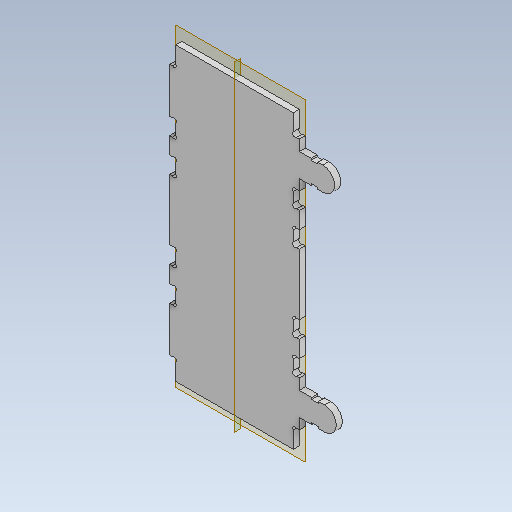
# Autodesk Inventor part: cover
Saved by Autodesk Inventor 2020 (Build 240168000, 168)
## iProperties
Created: 2019-12-17
Part Number: cover
Material: Generic
Document SubType Name: Modeling
Designer: erwin
Density: 1 g/cm^3
Appearance: Default
Author: erwin
Autodesk Inventor part; units mm, degrees
ref_plane "YZ Plane" through (0, 0, 0) normal (1, 0, 0) x (0, 1, 0)
ref_plane "XZ Plane" through (0, 0, 0) normal (0, 1, 0) x (-1, 0, 0)
ref_plane "XY Plane" through (0, 0, 0) normal (0, 0, 1) x (1, 0, 0)
ref_plane "Work Plane1" through (0, 0, 0) normal (0, 0, 1) x (1, 0, 0)
sketch "Sketch1" plane through (0, 0, 0) normal (0, 0, 1) x (1, 0, 0)
  line L0 (-35, -85) -> (-35, 85) projected
  line L1 (35, -85) -> (-35, -85) projected
  line L2 (35, 85) -> (35, -85) projected
  line L3 (-35, 85) -> (35, 85) projected
  line L4 (38.6, -88.6) -> (-38.6, -88.6)
  line L5 (-38.6, -88.6) -> (-38.6, 88.6)
  line L6 (-38.6, 88.6) -> (38.6, 88.6)
  line L7 (52.6163, 61.6) -> (37.6163, 61.6) construction
  arc A0 (52.6163, 54.6) -> (52.6163, 68.6) centre (52.6163, 61.6) ccw
  line L8 (38.6, -61.6) -> (53.6, -61.6) construction
  arc A1 (53.6, -68.6) -> (53.6, -54.6) centre (53.6, -61.6) ccw
  line L9 (38.6, 88.6) -> (38.6, 68.6)
  line L10 (38.6, 54.6) -> (38.6, -54.6)
  line L11 (38.6, -68.6) -> (38.6, -88.6)
  line L12 (45.6, 68.6) -> (45.6, 67.6)
  line L13 (45.6, 67.6) -> (49.6, 67.6)
  line L14 (49.6, 67.6) -> (49.6, 68.6)
  line L15 (49.6, 54.6) -> (49.6, 55.6)
  line L16 (49.6, 55.6) -> (45.6, 55.6)
  line L17 (45.6, 55.6) -> (45.6, 54.6)
  line L18 (38.6, 54.6) -> (45.6, 54.6)
  line L19 (49.6, 54.6) -> (52.6163, 54.6)
  line L20 (52.6163, 68.6) -> (49.6, 68.6)
  line L21 (45.6, 68.6) -> (38.6, 68.6)
  line L22 (49.9959, -54.6) -> (49.9945, -55.6)
  line L23 (49.9945, -55.6) -> (45.9945, -55.6)
  line L24 (45.9945, -55.6) -> (45.9959, -54.6)
  line L25 (49.9761, -68.6) -> (49.9736, -67.6)
  line L26 (49.9736, -67.6) -> (45.9736, -67.6)
  line L27 (45.9736, -67.6) -> (45.9761, -68.6)
  line L28 (53.6, -54.6) -> (49.9959, -54.6)
  line L29 (45.9959, -54.6) -> (38.6, -54.6)
  line L30 (38.6, -68.6) -> (45.9761, -68.6)
  line L31 (49.9761, -68.6) -> (53.6, -68.6)
  point P0 (0, 0)
  dimension "d1" = 7
  dimension "d2" = 7
  dimension "d7" = 4
  dimension "d8" = 1
  dimension "d9" = 7
  dimension "d10" = 15
  dimension "d11" = 15
  dimension "d12" = 3.6
  dimension "d13" = 3.6
  dimension "d14" = 1
  dimension "d15" = 1
  dimension "d16" = 20
  dimension "d17" = 20
  constraints: 60 end point, 14 parallel, 9 perpendicular, 8 tangent, 6 equal length, 5 point on circle, 3 collinear, 2 centre point, 2 point on line, 2 other
  measures "d1" radius of A0
  measures "d2" radius of A1
  measures "d7" distance of L12.end L13.end
  measures "d8" distance of L13.end L14.end
  measures "d9" distance between parallel lines of L9 L12
  measures "d10" distance of L7.start L7.end
  measures "d11" distance of L8.start L8.end
  measures "d12" distance between parallel lines of L2 L10
  measures "d13" distance between parallel lines of L6 L3
  measures "d14" distance of L22.start L22.end
  measures "d15" distance of L25.end L25.start
  measures "d16" distance between parallel lines of L4 L30
  measures "d17" distance between parallel lines of L6 L21
extrude "Extrusion1" add sketch "Sketch1" along normal blind 3.6 contours L0 L3 L2 L1 | L4 L5 L6 L9 L21 L12 L13 L14 L20 A0 L19 L15 L16 L17 L18 L10 L29 L24 L23 L22 L28 A1 L31 L25 L26 L27 L30 L11
sketch "Sketch2" plane through (0, 0, 0) normal (0, 0, -1) x (-1, 0, 0)
  line L0 (-49.6, 67.6) -> (-45.6, 67.6) projected
  line L1 (-49.6, 68.6) -> (-49.6, 67.6) projected
  line L2 (-52.6163, 68.6) -> (-49.6, 68.6) projected
  arc A0 (-52.6163, 68.6) -> (-52.6163, 54.6) centre (-52.6163, 61.6) ccw projected
  line L3 (-49.6, 54.6) -> (-52.6163, 54.6) projected
  line L4 (-49.6, 55.6) -> (-49.6, 54.6) projected
  line L5 (-45.6, 55.6) -> (-49.6, 55.6) projected
  line L6 (-45.6, 54.6) -> (-45.6, 55.6) projected
  line L7 (-38.6, 54.6) -> (-45.6, 54.6) projected
  line L8 (-38.6, -54.6) -> (-38.6, 54.6) projected
  line L9 (-45.9959, -54.6) -> (-38.6, -54.6) projected
  line L10 (-45.9945, -55.6) -> (-45.9959, -54.6) projected
  line L11 (-49.9945, -55.6) -> (-45.9945, -55.6) projected
  line L12 (-49.9959, -54.6) -> (-49.9945, -55.6) projected
  line L13 (-53.6, -54.6) -> (-49.9959, -54.6) projected
  arc A1 (-53.6, -54.6) -> (-53.6, -68.6) centre (-53.6, -61.6) ccw projected
  line L14 (-49.9761, -68.6) -> (-53.6, -68.6) projected
  line L15 (-49.9736, -67.6) -> (-49.9761, -68.6) projected
  line L16 (-45.9736, -67.6) -> (-49.9736, -67.6) projected
  line L17 (-45.9761, -68.6) -> (-45.9736, -67.6) projected
  line L18 (-38.6, -68.6) -> (-45.9761, -68.6) projected
  line L19 (-38.6, -88.6) -> (-38.6, -68.6) projected
  line L20 (38.6, -88.6) -> (-38.6, -88.6) projected
  line L21 (38.6, 88.6) -> (38.6, -88.6) projected
  line L22 (-38.6, 88.6) -> (38.6, 88.6) projected
  line L23 (-38.6, 68.6) -> (-38.6, 88.6) projected
  line L24 (-45.6, 68.6) -> (-38.6, 68.6) projected
  line L25 (-45.6, 67.6) -> (-45.6, 68.6) projected
  line L26 (35, -85) -> (35, 85) projected
  line L27 (35, 85) -> (-35, 85) projected
  line L28 (-35, 85) -> (-35, -85) projected
  line L29 (-35, -85) -> (35, -85) projected
  line L30 (38.6, 88.6) -> (38.6, -88.6) projected
  line L31 (-38.6, -88.6) -> (38.6, -88.6)
  line L32 (38.6, -88.6) -> (38.6, -85)
  line L33 (38.6, -85) -> (-38.6, -85)
  line L34 (-38.6, -85) -> (-38.6, -88.6)
  line L35 (-38.6, -85) -> (-35, -85)
  line L36 (-35, -85) -> (-35, -75)
  line L37 (-35, -75) -> (-38.6, -75)
  line L38 (-38.6, -75) -> (-38.6, -85)
  line L39 (-38.6, -54.6) -> (-38.6, 54.6) projected
  line L40 (-38.6, -48.2) -> (-35, -48.2)
  line L41 (-35, -48.2) -> (-35, -38.2)
  line L42 (-35, -38.2) -> (-38.6, -38.2)
  line L43 (-38.6, -38.2) -> (-38.6, -48.2)
  line L44 (-35, -28.2) -> (-38.6, -28.2)
  line L45 (-38.6, -28.2) -> (-38.6, -38.2)
  line L46 (-38.6, -38.2) -> (-35, -38.2)
  line L47 (-35, -38.2) -> (-35, -28.2)
  line L48 (-35, -18.2) -> (-38.6, -18.2)
  line L49 (-38.6, -18.2) -> (-38.6, -28.2)
  line L50 (-38.6, -28.2) -> (-35, -28.2)
  line L51 (-35, -28.2) -> (-35, -18.2)
  line L52 (-38.6, 0) -> (49.1643, 0) construction
  line L53 (-38.6, 88.6) -> (-38.6, 68.6)
  line L54 (38.6, 88.6) -> (-38.6, 88.6)
  line L55 (-35, 85) -> (35, 85)
  line L56 (-38.6, 88.6) -> (38.6, 88.6)
  line L57 (38.6, 88.6) -> (38.6, 85)
  line L58 (38.6, 85) -> (-38.6, 85)
  line L59 (-38.6, 85) -> (-38.6, 88.6)
  line L60 (-38.6, 85) -> (-35, 85)
  line L61 (-35, 85) -> (-35, 75)
  line L62 (-35, 75) -> (-38.6, 75)
  line L63 (-38.6, 75) -> (-38.6, 85)
  line L64 (-38.6, 48.2) -> (-35, 48.2)
  line L65 (-35, 48.2) -> (-35, 38.2)
  line L66 (-35, 38.2) -> (-38.6, 38.2)
  line L67 (-38.6, 38.2) -> (-38.6, 48.2)
  line L68 (-35, 28.2) -> (-38.6, 28.2)
  line L69 (-38.6, 28.2) -> (-38.6, 38.2)
  line L70 (-38.6, 38.2) -> (-35, 38.2)
  line L71 (-35, 38.2) -> (-35, 28.2)
  line L72 (-35, 18.2) -> (-38.6, 18.2)
  line L73 (-38.6, 18.2) -> (-38.6, 28.2)
  line L74 (-38.6, 28.2) -> (-35, 28.2)
  line L75 (-35, 28.2) -> (-35, 18.2)
  line L76 (38.6, -88.6) -> (-38.6, -88.6) construction
  line L77 (0, -88.6) -> (0, 88.6) construction
  line L78 (38.6, -54.6) -> (38.6, 54.6)
  line L79 (35, 85) -> (35, -85)
  line L80 (38.6, -85) -> (35, -85)
  line L81 (35, -85) -> (35, -75)
  line L82 (35, -75) -> (38.6, -75)
  line L83 (38.6, -75) -> (38.6, -85)
  line L84 (38.6, -54.6) -> (38.6, 54.6)
  line L85 (38.6, -48.2) -> (35, -48.2)
  line L86 (35, -48.2) -> (35, -38.2)
  line L87 (35, -38.2) -> (38.6, -38.2)
  line L88 (38.6, -38.2) -> (38.6, -48.2)
  line L89 (35, -28.2) -> (38.6, -28.2)
  line L90 (38.6, -28.2) -> (38.6, -38.2)
  line L91 (38.6, -38.2) -> (35, -38.2)
  line L92 (35, -38.2) -> (35, -28.2)
  line L93 (35, -18.2) -> (38.6, -18.2)
  line L94 (38.6, -18.2) -> (38.6, -28.2)
  line L95 (38.6, -28.2) -> (35, -28.2)
  line L96 (35, -28.2) -> (35, -18.2)
  line L97 (35, 18.2) -> (38.6, 18.2)
  line L98 (38.6, 18.2) -> (38.6, 28.2)
  line L99 (35, 28.2) -> (35, 18.2)
  line L100 (35, 28.2) -> (38.6, 28.2)
  line L101 (38.6, 28.2) -> (35, 28.2)
  line L102 (38.6, 28.2) -> (38.6, 38.2)
  line L103 (35, 38.2) -> (35, 28.2)
  line L104 (35, 38.2) -> (38.6, 38.2)
  line L105 (38.6, 38.2) -> (35, 38.2)
  line L106 (38.6, 48.2) -> (35, 48.2)
  line L107 (35, 48.2) -> (35, 38.2)
  line L108 (38.6, 85) -> (35, 85)
  line L109 (35, 85) -> (35, 75)
  line L110 (35, 75) -> (38.6, 75)
  line L111 (38.6, 38.2) -> (38.6, 48.2)
  line L112 (38.6, 75) -> (38.6, 85)
  point P0 (0, 0)
  point P1 (38.6, -68.6)
  point P2 (38.6, 68.6)
  point P3 (38.6, 0)
  dimension "d21" = 10
  dimension "d23" = 10
  dimension "d24" = 6.4
  dimension "d25" = 6.4
  dimension "d28" = 10
  constraints: 160 end point, 58 symmetric about line, 9 point on line, 6 parallel, 4 horizontal, 3 midpoint, 3 perpendicular, 1 vertical, 16 other
  measures "d21" distance of L36.end L35.end
  measures "d23" distance of L41.end L40.end
  measures "d24" distance between parallel lines of L37 L18
  measures "d25" distance between parallel lines of L9 L40
  measures "d28" distance of L41.end L44.start
extrude "Extrusion2" cut sketch "Sketch2" against normal through all contours L23 L58 L28 L62 | L23 L22 L21 L58 L27 | L28 L66 L8 L64 | L58 L21 L110 L26 | L28 L72 L8 L68 | L106 L21 L104 L26 | L28 L44 L8 L48 | L100 L21 L97 L26 | L28 L40 L8 L42 | L93 L21 L89 L26 | L28 L33 L19 L37 | L87 L21 L85 L26 | L29 L33 L21 L20 L19 | L26 L82 L21 L33
thicken "Thicken1" operation add thickness 1.8 both sides no extend neighbours yes toward (0, 1, 0) faces at (11.6667, 85, 2.4)
thicken "Thicken2" operation add thickness 1.8 both sides no extend neighbours yes toward (0, -1, 0) faces at (-11.6667, -85, 2.4)
sketch "Sketch3" plane through (0, 0, 3.6) normal (0, 0, 1) x (1, 0, 0)
  line L0 (38.6, -28.2) -> (35, -28.2) projected
  line L1 (35, -28.2) -> (35, -18.2) projected
  line L2 (35, -18.2) -> (38.6, -18.2) projected
  line L3 (38.6, -18.2) -> (38.6, 18.2) projected
  line L4 (38.6, 18.2) -> (35, 18.2) projected
  line L5 (35, 18.2) -> (35, 28.2) projected
  line L6 (35, 28.2) -> (38.6, 28.2) projected
  line L7 (38.6, 28.2) -> (38.6, 38.2) projected
  line L8 (38.6, 38.2) -> (35, 38.2) projected
  line L9 (35, 38.2) -> (35, 48.2) projected
  line L10 (35, 48.2) -> (38.6, 48.2) projected
  line L11 (38.6, 48.2) -> (38.6, 54.6) projected
  line L12 (38.6, 54.6) -> (45.6, 54.6) projected
  line L13 (45.6, 54.6) -> (45.6, 55.6) projected
  line L14 (45.6, 55.6) -> (49.6, 55.6) projected
  line L15 (49.6, 55.6) -> (49.6, 54.6) projected
  line L16 (49.6, 54.6) -> (52.6163, 54.6) projected
  arc A0 (52.6163, 54.6) -> (52.6163, 68.6) centre (52.6163, 61.6) ccw projected
  line L17 (52.6163, 68.6) -> (49.6, 68.6) projected
  line L18 (49.6, 68.6) -> (49.6, 67.6) projected
  line L19 (49.6, 67.6) -> (45.6, 67.6) projected
  line L20 (45.6, 67.6) -> (45.6, 68.6) projected
  line L21 (45.6, 68.6) -> (38.6, 68.6) projected
  line L22 (38.6, 68.6) -> (38.6, 75) projected
  line L23 (38.6, 75) -> (35, 75) projected
  line L24 (35, 75) -> (35, 86.8) projected
  line L25 (35, 86.8) -> (-35, 86.8) projected
  line L26 (-35, 86.8) -> (-35, 75) projected
  line L27 (-35, 75) -> (-38.6, 75) projected
  line L28 (-38.6, 75) -> (-38.6, 48.2) projected
  line L29 (-38.6, 48.2) -> (-35, 48.2) projected
  line L30 (-35, 48.2) -> (-35, 38.2) projected
  line L31 (-35, 38.2) -> (-38.6, 38.2) projected
  line L32 (-38.6, 38.2) -> (-38.6, 28.2) projected
  line L33 (-38.6, 28.2) -> (-35, 28.2) projected
  line L34 (-35, 28.2) -> (-35, 18.2) projected
  line L35 (-35, 18.2) -> (-38.6, 18.2) projected
  line L36 (-38.6, 18.2) -> (-38.6, -18.2) projected
  line L37 (-38.6, -18.2) -> (-35, -18.2) projected
  line L38 (-35, -18.2) -> (-35, -28.2) projected
  line L39 (-35, -28.2) -> (-38.6, -28.2) projected
  line L40 (-38.6, -28.2) -> (-38.6, -38.2) projected
  line L41 (-38.6, -38.2) -> (-35, -38.2) projected
  line L42 (-35, -38.2) -> (-35, -48.2) projected
  line L43 (-35, -48.2) -> (-38.6, -48.2) projected
  line L44 (-38.6, -48.2) -> (-38.6, -75) projected
  line L45 (-38.6, -75) -> (-35, -75) projected
  line L46 (-35, -75) -> (-35, -86.8) projected
  line L47 (-35, -86.8) -> (35, -86.8) projected
  line L48 (35, -86.8) -> (35, -75) projected
  line L49 (35, -75) -> (38.6, -75) projected
  line L50 (38.6, -75) -> (38.6, -68.6) projected
  line L51 (38.6, -68.6) -> (45.9761, -68.6) projected
  line L52 (45.9761, -68.6) -> (45.9736, -67.6) projected
  line L53 (45.9736, -67.6) -> (49.9736, -67.6) projected
  line L54 (49.9736, -67.6) -> (49.9761, -68.6) projected
  line L55 (49.9761, -68.6) -> (53.6, -68.6) projected
  arc A1 (53.6, -68.6) -> (53.6, -54.6) centre (53.6, -61.6) ccw projected
  line L56 (53.6, -54.6) -> (49.9959, -54.6) projected
  line L57 (49.9959, -54.6) -> (49.9945, -55.6) projected
  line L58 (49.9945, -55.6) -> (45.9945, -55.6) projected
  line L59 (45.9945, -55.6) -> (45.9959, -54.6) projected
  line L60 (45.9959, -54.6) -> (38.6, -54.6) projected
  line L61 (38.6, -54.6) -> (38.6, -48.2) projected
  line L62 (38.6, -48.2) -> (35, -48.2) projected
  line L63 (35, -48.2) -> (35, -38.2) projected
  line L64 (35, -38.2) -> (38.6, -38.2) projected
  line L65 (38.6, -38.2) -> (38.6, -28.2) projected
  circle A2 centre (-35.9899, 75.9899) radius 1.4
  line L66 (-36.9799, 75) -> (-35, 75) construction
  line L67 (-35, 75) -> (-35, 76.9799) construction
  line L68 (-35, 76.9799) -> (-36.9799, 76.9799) construction
  line L69 (-36.9799, 76.9799) -> (-36.9799, 75) construction
  line L70 (-36.9799, 75) -> (-35, 76.9799) construction
  line L71 (-35, 75) -> (-36.9799, 76.9799) construction
  circle A3 centre (-35.9899, 47.2101) radius 1.4
  line L72 (-36.9799, 46.2201) -> (-35, 46.2201) construction
  line L73 (-35, 46.2201) -> (-35, 48.2) construction
  line L74 (-35, 48.2) -> (-36.9799, 48.2) construction
  line L75 (-36.9799, 48.2) -> (-36.9799, 46.2201) construction
  line L76 (-36.9799, 46.2201) -> (-35, 48.2) construction
  line L77 (-35, 46.2201) -> (-36.9799, 48.2) construction
  circle A4 centre (-35.9899, 39.1899) radius 1.4
  line L78 (-36.9799, 38.2) -> (-35, 38.2) construction
  line L79 (-35, 38.2) -> (-35, 40.1799) construction
  line L80 (-35, 40.1799) -> (-36.9799, 40.1799) construction
  line L81 (-36.9799, 40.1799) -> (-36.9799, 38.2) construction
  line L82 (-36.9799, 38.2) -> (-35, 40.1799) construction
  line L83 (-35, 38.2) -> (-36.9799, 40.1799) construction
  line L84 (-36.9799, 26.2201) -> (-35, 26.2201) construction
  circle A5 centre (-35.9899, 27.2101) radius 1.4
  line L85 (-36.9799, 28.2) -> (-36.9799, 26.2201) construction
  line L86 (-36.9799, 26.2201) -> (-35, 28.2) construction
  line L87 (-35, 26.2201) -> (-36.9799, 28.2) construction
  line L88 (-35, 28.2) -> (-36.9799, 28.2) construction
  line L89 (-35, 26.2201) -> (-35, 28.2) construction
  line L90 (-36.9799, 18.2) -> (-35, 18.2) construction
  circle A6 centre (-35.9899, 19.1899) radius 1.4
  line L91 (-36.9799, 20.1799) -> (-36.9799, 18.2) construction
  line L92 (-36.9799, 18.2) -> (-35, 20.1799) construction
  line L93 (-35, 18.2) -> (-36.9799, 20.1799) construction
  line L94 (-35, 20.1799) -> (-36.9799, 20.1799) construction
  line L95 (-35, 18.2) -> (-35, 20.1799) construction
  line L96 (-36.9799, -40.1799) -> (-35, -40.1799) construction
  circle A7 centre (-35.9899, -39.1899) radius 1.4
  line L97 (-36.9799, -38.2) -> (-36.9799, -40.1799) construction
  line L98 (-36.9799, -40.1799) -> (-35, -38.2) construction
  line L99 (-35, -40.1799) -> (-36.9799, -38.2) construction
  line L100 (-35, -38.2) -> (-36.9799, -38.2) construction
  line L101 (-35, -40.1799) -> (-35, -38.2) construction
  line L102 (-36.9799, -48.2) -> (-35, -48.2) construction
  circle A8 centre (-35.9899, -47.2101) radius 1.4
  line L103 (-36.9799, -46.2201) -> (-36.9799, -48.2) construction
  line L104 (-36.9799, -48.2) -> (-35, -46.2201) construction
  line L105 (-35, -48.2) -> (-36.9799, -46.2201) construction
  line L106 (-35, -46.2201) -> (-36.9799, -46.2201) construction
  line L107 (-35, -48.2) -> (-35, -46.2201) construction
  line L108 (-36.9799, -20.1799) -> (-35, -20.1799) construction
  circle A9 centre (-35.9899, -19.1899) radius 1.4
  line L109 (-36.9799, -18.2) -> (-36.9799, -20.1799) construction
  line L110 (-36.9799, -20.1799) -> (-35, -18.2) construction
  line L111 (-35, -20.1799) -> (-36.9799, -18.2) construction
  line L112 (-35, -18.2) -> (-36.9799, -18.2) construction
  line L113 (-35, -20.1799) -> (-35, -18.2) construction
  line L114 (-36.9799, -28.2) -> (-35, -28.2) construction
  circle A10 centre (-35.9899, -27.2101) radius 1.4
  line L115 (-36.9799, -26.2201) -> (-36.9799, -28.2) construction
  line L116 (-36.9799, -28.2) -> (-35, -26.2201) construction
  line L117 (-35, -28.2) -> (-36.9799, -26.2201) construction
  line L118 (-35, -26.2201) -> (-36.9799, -26.2201) construction
  line L119 (-35, -28.2) -> (-35, -26.2201) construction
  line L120 (-36.9799, -76.9799) -> (-35, -76.9799) construction
  circle A11 centre (-35.9899, -75.9899) radius 1.4
  line L121 (-36.9799, -75) -> (-36.9799, -76.9799) construction
  line L122 (-36.9799, -76.9799) -> (-35, -75) construction
  line L123 (-35, -76.9799) -> (-36.9799, -75) construction
  line L124 (-35, -75) -> (-36.9799, -75) construction
  line L125 (-35, -76.9799) -> (-35, -75) construction
  point P0 (0, 0)
  dimension "d40" = 2.8
  dimension "d42" = 2.8
  dimension "d44" = 2.8
  dimension "d46" = 2.8
  dimension "d47" = 2.8
  dimension "d50" = 2.8
  dimension "d51" = 2.8
  dimension "d54" = 2.8
  dimension "d55" = 2.8
  dimension "d58" = 2.8
  constraints: 120 end point, 20 midpoint, 20 parallel, 20 perpendicular, 10 horizontal, 30 other
ref_plane "Work Plane2" through (0, -18.2, 0) normal (-1, 0, 0) x (0, 0, 1)
extrude "Extrusion3" cut sketch "Sketch3" against normal through all contours A11 L45 L46 | L46 A11 | L45 A11 | A8 L42 L43 | L43 A8 | L42 A8 | A7 L41 L42 | L42 A7 | A2 L26 | L26 L27 A2 | L41 A7 | A2 L27 | A10 L38 L39 | L39 A10 | A3 L29 | L29 L30 A3 | L38 A10 | A3 L30 | A9 L37 L38 | L38 A9 | A4 L30 | L30 L31 A4 | L37 A9 | A4 L31 | A6 L34 L35 | L35 A6 | A5 L33 | L33 L34 A5 | L34 A6 | A5 L34
mirror "Mirror1" about plane through (0, -18.2, 0) normal (-1, 0, 0) of "Extrusion3"
equation "\"d2\" = d1"
equation "\"d11\" = d10"
equation "\"d12\" = wood_thickness"
equation "\"d13\" = d12"
equation "\"d14\" = d8"
equation "\"d15\" = d8"
equation "\"d16\" = d17"
equation "\"d18\" = wood_thickness"
equation "\"d21\" = tabs_width"
equation "\"d23\" = tabs_width"
equation "\"d25\" = d24"
equation "\"d28\" = tabs_width"
equation "\"d35\" = deep_for_sliding_cover"
equation "\"d36\" = deep_for_sliding_cover"
equation "\"d37\" = deep_for_sliding_cover"
equation "\"d38\" = deep_for_sliding_cover"
equation "\"d40\" = d41"
equation "\"d42\" = d43"
equation "\"d44\" = d45"
equation "\"d46\" = d48"
equation "\"d47\" = d49"
equation "\"d50\" = d52"
equation "\"d51\" = d53"
equation "\"d54\" = d56"
equation "\"d55\" = d57"
equation "\"d58\" = d60"
equation "\"d0\" = wood_thickness"
equation "\"wood_thickness\" = 3.6"
equation "\"tabs_width\" = 10"
equation "\"deep_for_sliding_cover\" = 1.8"
equation "\"d41\" = 2.8"
equation "\"d43\" = 2.8"
equation "\"d45\" = 2.8"
equation "\"d48\" = 2.8"
equation "\"d49\" = 2.8"
equation "\"d52\" = 2.8"
equation "\"d53\" = 2.8"
equation "\"d56\" = 2.8"
equation "\"d57\" = 2.8"
equation "\"d60\" = 2.8"
body "Solid1"
